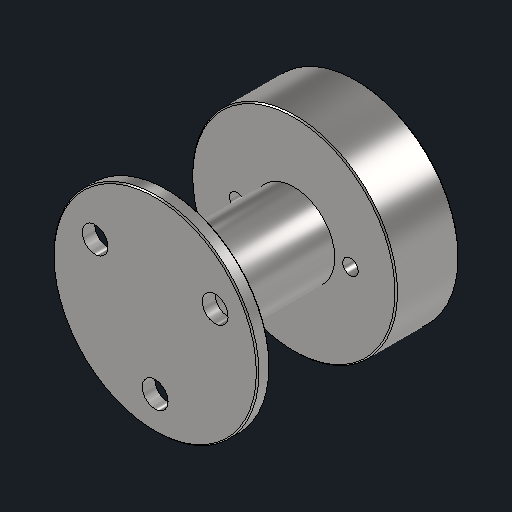
# Autodesk Inventor part: HayashiProbeHead
Saved by Autodesk Inventor 2027.1 (Build 311270010, 270A)
## iProperties
Created: 2025-06-19
Part Number: HayashiProbeHead
Material: Stainless Steel
Document SubType Name: Modeling
Designer: kuzmin
Density: 8 g/cm^3
Appearance: Semi-Polished
Author: kuzmin
Autodesk Inventor part; units mm, degrees
note: some values were not read from the file. Chosen so that the rebuilt part matches the saved one: direction of "Hole3".
ref_plane "YZ Plane" through (0, 0, 0) normal (1, 0, 0) x (0, 1, 0)
ref_plane "XZ Plane" through (0, 0, 0) normal (0, 1, 0) x (-1, 0, 0)
ref_plane "XY Plane" through (0, 0, 0) normal (0, 0, 1) x (1, 0, 0)
sketch "Sketch1" plane through (0, 0, 0) normal (0, 1, 0) x (-1, 0, 0)
  line L0 (6.5, -2) -> (6.5, -22)
  line L1 (16.25, -22) -> (16.25, -32)
  line L2 (16.25, 0) -> (16.25, -2)
  line L3 (0, 0) -> (0, -32)
  line L4 (16.25, 0) -> (0, 0)
  line L5 (16.25, -2) -> (6.5, -2)
  line L6 (16.25, -22) -> (6.5, -22)
  line L7 (16.25, -32) -> (0, -32)
  point P0 (0, 26.9125)
  point P1 (0, -16.1673)
  point P2 (0, 6.9125)
  point P3 (0, -16)
  dimension "d19" = 20
  dimension "d20" = 10
  dimension "d21" = 2
  dimension "d22" = 32.5
  dimension "d23" = 13
  dimension "d24" = 32.5
  constraints: 16 end point, 3 parallel, 3 vertical alignment, 1 coincident, 1 horizontal, 1 midpoint, 1 vertical
  measures "d19" distance of L0.start L0.end
  measures "d20" distance of L1.start L1.end
  measures "d21" distance of L2.start L2.end
  measures "d22" diameter of L1 L3
  measures "d23" diameter of L0 L3
  measures "d24" diameter of L2 L3
revolve "Revolution1" add sketch "Sketch1" angle 360 about axis through (0, 0, 0) along (0, 0, -1)
sketch "Sketch3" plane through (0, 0, -2) normal (0, 0, -1) x (-1, 0, 0)
  circle A0 centre (0, 0) radius 11 construction
  point P0 (0, -11)
  dimension "d25" = 22
  constraints: 1 coincident, 1 vertical alignment, 2 other
hole "Hole2" at (0, -11, -2) direction (0, 0, 1) diameter 4.1 end through all
pattern_circular "Circular Pattern2" count 3 over 360 about axis through (0, 0, -10) along (0, 0, 1) of "Hole2"
sketch "Sketch4" plane through (0, 0, -32) normal (0, 0, -1) x (-1, 0, 0)
  line L0 (9, 0) -> (-9, 0) construction
  point P0 (0, 0)
  point P1 (0, 0)
  dimension "d36" = 18
  constraints: 3 coincident, 2 end point, 1 horizontal, 1 midpoint
  measures "d36" distance of L0.start L0.end
hole "Hole3" at (-9, 0, -32) at (9, 0, -32) direction (0, 0, 1) diameter 2.459 depth 10 thread size "M3x0.5" class "6H" standard "ANSI Metric M Profile"
chamfer "Chamfer1" distance 0.2 angle 45 4 edges at (16.25, 0, -32) (16.25, 0, -22) (16.25, 0, -2) (16.25, 0, 0)
equation "\"d23\" = stockid"
equation "\"d25\" = holesid"
equation "\"holesid\" = 22"
equation "\"stockid\" = 13"
body "Solid1"
